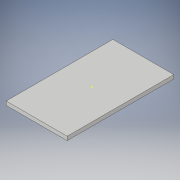
# Autodesk Inventor part: caseing
Saved by Autodesk Inventor 2019 (Build 230136000, 136)
## iProperties
Created: 2020-02-18
Part Number: caseing
Material: Generic
Document SubType Name: Modeling
Designer: Lenovo
Density: 1 g/cm^3
Appearance: Default
Author: Lenovo
Autodesk Inventor part; units mm, degrees
ref_plane "YZ Plane" through (0, 0, 0) normal (1, 0, 0) x (0, 1, 0)
ref_plane "XZ Plane" through (0, 0, 0) normal (0, 1, 0) x (-1, 0, 0)
ref_plane "XY Plane" through (0, 0, 0) normal (0, 0, 1) x (1, 0, 0)
sketch "Sketch1" plane through (0, 0, 0) normal (0, 1, 0) x (-1, 0, 0)
  line L0 (9, 18) -> (-7, 18)
  line L1 (-7, 18) -> (-7, -10)
  line L2 (-7, -10) -> (9, -10)
  line L3 (9, -10) -> (9, 18)
  point P0 (0, 0)
  constraints: 8 end point, 2 parallel, 1 horizontal, 1 perpendicular
extrude "Extrusion1" add sketch "Sketch1" along normal blind 1
sketch "Sketch2" plane through (0, 1, 0) normal (0, 1, 0) x (1, 0, 0)
  point P0 (0, 0)
scale "Scale1" factors (10, 10, 10) then translate (9, -9, -36) bodies 1
scale "Scale2" factors (10, 10, 10) then translate (9, -9, -36) bodies 1
scale "Scale3" factors (0.1, 0.1, 0.1) then translate (-0.9, 0.9, 3.6) bodies 1
body "Solid1"
